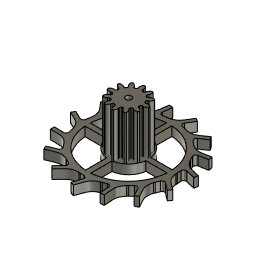
EscapeWheel v5 (Autodesk Fusion 360 design; units mm, degrees)
description: Spur Gear; Module: 2.0; Num Teeth: 12; Pressure Angle: 20.0; Backlash: 0.10 mm
Autodesk Fusion 360 part; units mm, degrees
sketch "main" plane through (0, 0, 0) normal (0, 0, 1) x (1, 0, 0) in component "Spur Gear (12 teeth)"
  circle A0 centre (0, 0) radius 9.5492
  circle A1 centre (0, 0) radius 2.25
extrude "Extrude1" add sketch "main" along normal blind 40 makes body 1 in component "Spur Gear (12 teeth)"
sketch "pin" plane through (0, 0, 0) normal (0, 0, 1) x (1, 0, 0) in component "Spur Gear (12 teeth)"
  spline S0 degree 5 poles (11.1601, -1.6151) (11.1681, -1.6162) (11.1841, -1.6183) (11.2082, -1.6206) (11.2404, -1.6222) (11.2808, -1.6223) (11.3214, -1.6209) (11.3621, -1.6186) (11.4028, -1.6159) (11.4435, -1.6128) (11.4843, -1.6094) (11.5251, -1.6055) (11.566, -1.6009) (11.6069, -1.5957) (11.6478, -1.5898) (11.6887, -1.5832) (11.7297, -1.576) (11.7707, -1.5684) (11.8117, -1.5604) (11.8527, -1.5519) (11.8937, -1.5431) (11.9347, -1.5338) (11.9757, -1.5241) (12.0167, -1.514) (12.0577, -1.5034) (12.0987, -1.4923) (12.1397, -1.4809) (12.1807, -1.469) (12.2216, -1.4568) (12.2626, -1.4443) (12.3035, -1.4313) (12.3444, -1.418) (12.3853, -1.4043) (12.4262, -1.3902) (12.467, -1.3758) (12.5079, -1.361) (12.5487, -1.3459) (12.5894, -1.3304) (12.6302, -1.3146) (12.6709, -1.2984) (12.7115, -1.282) (12.7522, -1.2651) (12.7928, -1.248) (12.8334, -1.2305) (12.8739, -1.2127) (12.9144, -1.1946) (12.9548, -1.1761) (12.9952, -1.1573) (13.0356, -1.1383) (13.0759, -1.1189) (13.1161, -1.0992) (13.1564, -1.0792) (13.1965, -1.0589) (13.2366, -1.0382) (13.2767, -1.0173) (13.3167, -0.9961) (13.3567, -0.9746) (13.3966, -0.9528) (13.4364, -0.9307) (13.4762, -0.9083) (13.5159, -0.8857) (13.5556, -0.8627) (13.5952, -0.8394) (13.6347, -0.8159) (13.6742, -0.7921) (13.7136, -0.768) (13.7529, -0.7436) (13.7922, -0.719) (13.8314, -0.6941) (13.8705, -0.6689) (13.9096, -0.6434) (13.9408, -0.6228) (13.9642, -0.6072) (13.9797, -0.5968) (13.9875, -0.5916) knots 0 0 0 0 0 0 0.01428571 0.02857143 0.04285714 0.05714286 0.07142857 0.08571429 0.1 0.11428571 0.12857143 0.14285714 0.15714286 0.17142857 0.18571429 0.2 0.21428571 0.22857143 0.24285714 0.25714286 0.27142857 0.28571429 0.3 0.31428571 0.32857143 0.34285714 0.35714286 0.37142857 0.38571429 0.4 0.41428571 0.42857143 0.44285714 0.45714286 0.47142857 0.48571429 0.5 0.51428571 0.52857143 0.54285714 0.55714286 0.57142857 0.58571429 0.6 0.61428571 0.62857143 0.64285714 0.65714286 0.67142857 0.68571429 0.7 0.71428571 0.72857143 0.74285714 0.75714286 0.77142857 0.78571429 0.8 0.81428571 0.82857143 0.84285714 0.85714286 0.87142857 0.88571429 0.9 0.91428571 0.92857143 0.94285714 0.95714286 0.97142857 0.98571429 1 1 1 1 1 1
  spline S1 degree 5 poles (11.1601, 1.6151) (11.1681, 1.6162) (11.1841, 1.6183) (11.2082, 1.6206) (11.2404, 1.6222) (11.2808, 1.6223) (11.3214, 1.6209) (11.3621, 1.6186) (11.4028, 1.6159) (11.4435, 1.6128) (11.4843, 1.6094) (11.5251, 1.6055) (11.566, 1.6009) (11.6069, 1.5957) (11.6478, 1.5898) (11.6887, 1.5832) (11.7297, 1.576) (11.7707, 1.5684) (11.8117, 1.5604) (11.8527, 1.5519) (11.8937, 1.5431) (11.9347, 1.5338) (11.9757, 1.5241) (12.0167, 1.514) (12.0577, 1.5034) (12.0987, 1.4923) (12.1397, 1.4809) (12.1807, 1.469) (12.2216, 1.4568) (12.2626, 1.4443) (12.3035, 1.4313) (12.3444, 1.418) (12.3853, 1.4043) (12.4262, 1.3902) (12.467, 1.3758) (12.5079, 1.361) (12.5487, 1.3459) (12.5894, 1.3304) (12.6302, 1.3146) (12.6709, 1.2984) (12.7115, 1.282) (12.7522, 1.2651) (12.7928, 1.248) (12.8334, 1.2305) (12.8739, 1.2127) (12.9144, 1.1946) (12.9548, 1.1761) (12.9952, 1.1573) (13.0356, 1.1383) (13.0759, 1.1189) (13.1161, 1.0992) (13.1564, 1.0792) (13.1965, 1.0589) (13.2366, 1.0382) (13.2767, 1.0173) (13.3167, 0.9961) (13.3567, 0.9746) (13.3966, 0.9528) (13.4364, 0.9307) (13.4762, 0.9083) (13.5159, 0.8857) (13.5556, 0.8627) (13.5952, 0.8394) (13.6347, 0.8159) (13.6742, 0.7921) (13.7136, 0.768) (13.7529, 0.7436) (13.7922, 0.719) (13.8314, 0.6941) (13.8705, 0.6689) (13.9096, 0.6434) (13.9408, 0.6228) (13.9642, 0.6072) (13.9797, 0.5968) (13.9875, 0.5916) knots 0 0 0 0 0 0 0.01428571 0.02857143 0.04285714 0.05714286 0.07142857 0.08571429 0.1 0.11428571 0.12857143 0.14285714 0.15714286 0.17142857 0.18571429 0.2 0.21428571 0.22857143 0.24285714 0.25714286 0.27142857 0.28571429 0.3 0.31428571 0.32857143 0.34285714 0.35714286 0.37142857 0.38571429 0.4 0.41428571 0.42857143 0.44285714 0.45714286 0.47142857 0.48571429 0.5 0.51428571 0.52857143 0.54285714 0.55714286 0.57142857 0.58571429 0.6 0.61428571 0.62857143 0.64285714 0.65714286 0.67142857 0.68571429 0.7 0.71428571 0.72857143 0.74285714 0.75714286 0.77142857 0.78571429 0.8 0.81428571 0.82857143 0.84285714 0.85714286 0.87142857 0.88571429 0.9 0.91428571 0.92857143 0.94285714 0.95714286 0.97142857 0.98571429 1 1 1 1 1 1
  arc A0 (13.9875, -0.5916) -> (13.9875, 0.5916) centre (0, 0) ccw
  line L0 (9.4409, -1.3677) -> (11.1601, -1.6151)
  line L1 (9.4409, 1.3677) -> (11.1601, 1.6151)
  line L2 (9.4409, -1.3677) -> (9.4409, 1.3677)
  point P0 (11.3561, -1.6189)
  point P1 (11.5549, -1.6021)
  point P2 (11.7554, -1.5712)
  point P3 (11.9572, -1.5284)
  point P4 (12.1599, -1.475)
  point P5 (12.3633, -1.4116)
  point P6 (12.567, -1.3389)
  point P7 (12.771, -1.2571)
  point P8 (12.9749, -1.1667)
  point P9 (13.1786, -1.0679)
  point P10 (13.3819, -0.9608)
  point P11 (13.5846, -0.8456)
  point P12 (13.7865, -0.7225)
  point P13 (11.3561, 1.6189)
  point P14 (11.5549, 1.6021)
  point P15 (11.7554, 1.5712)
  point P16 (11.9572, 1.5284)
  point P17 (12.1599, 1.475)
  point P18 (12.3633, 1.4116)
  point P19 (12.567, 1.3389)
  point P20 (12.771, 1.2571)
  point P21 (12.9749, 1.1667)
  point P22 (13.1786, 1.0679)
  point P23 (13.3819, 0.9608)
  point P24 (13.5846, 0.8456)
  point P25 (13.7865, 0.7225)
extrude "Extrude2" add sketch "pin" along normal blind 40 bodies 1 in component "Spur Gear (12 teeth)"
fillet "Fillet1" radius 0.8 2 edges at (9.4505, -1.3691, 20) (9.4505, 1.3691, 20) on bodies 1 in component "Spur Gear (12 teeth)"
pattern_circular "C-Pattern1" count 12 over 360 about axis through (0, 0, 0) along (0, 0, 1) of "Extrude2", "Fillet1" in component "Spur Gear (12 teeth)"
sketch "area" plane through (0, 0, 0) normal (0, 0, 1) x (1, 0, 0) in component "Spur Gear (12 teeth)"
  circle A0 centre (0, 0) radius 12 construction
sketch "base" plane through (0, 0, 0) normal (0, 0, 1) x (1, 0, 0)
  circle A0 centre (0, 0) radius 35
  line L0 (-2.1738, 14.8417) -> (-2.1738, 30.9237)
  line L1 (1.8319, 14.8877) -> (1.8319, 30.9458)
  line L2 (-14.8877, 1.8319) -> (-30.9458, 1.8319)
  line L3 (-14.8417, -2.1738) -> (-30.9237, -2.1738)
  line L4 (-1.8319, -14.8877) -> (-1.8319, -30.9458)
  line L5 (2.1738, -14.8417) -> (2.1738, -30.9237)
  line L6 (14.8877, -1.8319) -> (30.9458, -1.8319)
  line L7 (14.8417, 2.1738) -> (30.9237, 2.1738)
  arc A1 (14.8417, 2.1738) -> (1.8319, 14.8877) centre (0, 0) ccw
  arc A2 (30.9237, 2.1738) -> (1.8319, 30.9458) centre (0, 0) ccw
  arc A3 (2.1738, -14.8417) -> (14.8877, -1.8319) centre (0, 0) ccw
  arc A4 (2.1738, -30.9237) -> (30.9458, -1.8319) centre (0, 0) ccw
  arc A5 (-2.1738, 14.8417) -> (-14.8877, 1.8319) centre (0, 0) ccw
  arc A6 (-14.8417, -2.1738) -> (-1.8319, -14.8877) centre (0, 0) ccw
  arc A7 (-2.1738, 30.9237) -> (-30.9458, 1.8319) centre (0, 0) ccw
  arc A8 (-30.9237, -2.1738) -> (-1.8319, -30.9458) centre (0, 0) ccw
  line L8 (6.1104, 34.5914) -> (14.4686, 32.369)
  line L9 (4.9262, 37.5808) -> (8.6182, 43.5145)
  arc A9 (4.9262, 37.5808) -> (6.1104, 34.5914) centre (6.6244, 36.5242) ccw
  line L10 (8.6182, 43.5145) -> (6.071, 45.0994)
  spline S0 degree 5 poles (6.071, 45.0994) (5.9212, 44.8332) (5.6229, 44.3065) (5.1798, 43.5337) (4.599, 42.5405) (3.8977, 41.3783) (3.2319, 40.3174) (2.6119, 39.3798) (2.0459, 38.5835) (1.5369, 37.9362) (1.0807, 37.4317) (0.6628, 37.0425) (0.2619, 36.7298) (-0.1453, 36.4542) (-0.5801, 36.1855) (-1.0577, 35.9129) (-1.5881, 35.6393) (-2.1778, 35.3747) (-2.8301, 35.1306) (-3.4199, 34.9523) (-3.8976, 34.8325) (-4.2363, 34.7584) (-4.419, 34.7213) (-4.4382, 34.7175) knots 0 0 0 0 0 0 0.05 0.1 0.15 0.2 0.25 0.3 0.35 0.4 0.45 0.5 0.55 0.6 0.65 0.7 0.75 0.8 0.85 0.9 0.90585 0.90585 0.90585 0.90585 0.90585 0.90585
  line L11 (7.1423, 47.0026) -> (4.9998, 43.1962)
  line L12 (-2.5645, 35.0944) -> (-6.3119, 34.3405)
  circle A10 centre (0, 0) radius 2.25
  point P0 (1.5101, 37.9244)
  point P1 (-0.1518, 36.4563)
  point P2 (-2.1692, 35.3897)
  dimension "d8" = 30
  dimension "d9" = 62
  dimension "d10" = 70
  dimension "d12" = 360
  dimension "d15" = 73
  dimension "d16" = 2
  dimension "d17" = 3
  dimension "d24" = 4.5
  constraint coincident A0.centre A1.centre
  constraint vertical L0
  constraint vertical L1
  constraint concentric A1 A5
  constraint concentric A2 A7
  constraint concentric A3 A5
  constraint concentric A4 A7
  constraint concentric A5 A6
  constraint concentric A7 A8
  constraint tangent A0 L8
  constraint tangent L8 A9
  constraint tangent L9 A9
  constraint perpendicular L9 L10
  constraint coincident A0 S0.end
  constraint midpoint L10.end L11
  constraint midpoint S0.end L12
  constraint concentric A4 A10
  measures "d8" diameter of A5
  measures "d9" diameter of A7
  measures "d10" diameter of A0
  measures "d15" angle of L8 L9
  measures "d16" radius of A9
  measures "d17" distance of L9.end L10.end
  measures "d24" diameter of A10
extrude "Extrude1'" add sketch "base" along normal blind 7 separate body contours A0 L8 L9 A9 L10 S0 makes body 2
pattern_circular "C-Pattern1'" count 15 over 360 about axis through (0, 0, 0) along (0, 0, 1) of "Extrude1'" makes body 3 makes body 4 makes body 5 makes body 6 makes body 7 makes body 8 makes body 9 makes body 10 makes body 11 makes body 12 makes body 13 makes body 14 makes body 15 makes body 16
extrude "Extrude2'" add sketch "base" along normal blind 7 contours A0 | A10 bodies 2 3 4 5 6 7 8 9 10 11 12 13 14 15 16
extrude "Extrude3" cut sketch "base" along normal blind 22 contours A10 bodies 2
copy_body "Body->Comp1" bodies 2 removing the originals makes body 17 in component "EscapeWheel"
component "Spur Gear (12 teeth)" placed x (0.991445, 0.130526, 0) y (-0.130526, 0.991445, 0) z (0, 0, 1) at (0, 0, 0)
component "EscapeWheel" placed x (1, 0, 0) y (0, 1, 0) z (0, 0, 1) at (0, 0, 0)
named bodies: "Gear12", "EscapeWheel"
